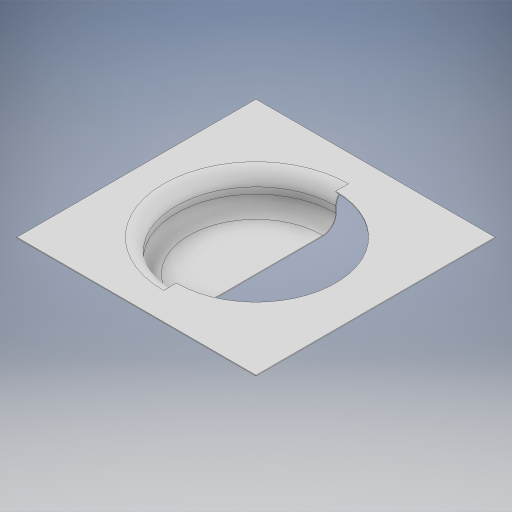
# Autodesk Inventor part: A3.2
Saved by Autodesk Inventor 2024 (Build 280153000, 153)
## iProperties
Created: 2024-03-14
Part Number: A3.2
Material: Generic
Document SubType Name: Sheet Metal
Designer: Alex
Density: 1 g/cm^3
Sheet Metal Rule: Default_mm
Appearance: Default
Author: Alex
Autodesk Inventor part; units mm, degrees
ref_plane "YZ Plane" through (0, 0, 0) normal (1, 0, 0) x (0, 1, 0)
ref_plane "XZ Plane" through (0, 0, 0) normal (0, 1, 0) x (-1, 0, 0)
sketch "Sketch1" plane through (0, 0, 0) normal (0, 1, 0) x (-1, 0, 0)
  line L0 (0, 0) -> (-150, 0)
  line L1 (-150, 0) -> (-150, -150)
  line L2 (-150, -150) -> (0, -150)
  line L3 (0, -150) -> (0, 0)
  dimension "d0" = 150
  dimension "d1" = 150
  measures "d0" distance of L2.end L1.end
  measures "d1" distance of L1.end L0.end
extrude "Plate1" add sketch "Sketch1" along normal blind 0.5
sketch "Sketch2" plane through (0, 0.5, 0) normal (0, 1, 0) x (1, 0, 0)
  arc A0 (75, 133) -> (75, 17) centre (75, 75) ccw
  line L0 (0, 0) -> (0, 150) projected
  line L1 (0, 150) -> (150, 150) projected
  line L2 (75, 17) -> (75, 133) construction
  arc A1 (75, 25) -> (75, 125) centre (75, 75) ccw
  line L3 (75, 125) -> (75, 133)
  line L4 (75, 25) -> (75, 17)
  arc A2 (75, 17) -> (75, 133) centre (75, 75) ccw construction
  dimension "d3" = 75
  dimension "d4" = 75
  dimension "d5" = 116
  dimension "d7" = 50
  constraints: 6 end point, 6 point on circle, 3 centre point, 2 coincident, 2 collinear, 2 point on line, 1 midpoint, 1 vertical
  measures "d3" distance from line of L0 A0.centre
  measures "d4" distance from line of L1 A0.centre
  measures "d5" diameter of A0
  measures "d7" radius of A1
extrude "Extrusion1" cut sketch "Sketch2" against normal blind 0.5
ref_plane "Work Plane1" through (75, 0.5, -75) normal (0, 0, -1) x (-1, 0, 0)
sketch "Sketch3" plane through (75, 0.5, -75) normal (0, 0, -1) x (-1, 0, 0)
  line L0 (58, 0) -> (0, 0) construction
  line L1 (0, 0) -> (0, -0.5) projected
  line L2 (0, 0) -> (0, -20)
  line L3 (0, -20) -> (42, -20)
  arc A0 (42, -20) -> (50, -12) centre (42, -12) ccw
  line L4 (50, -12) -> (50, -8)
  arc A1 (58, 0) -> (50, -8) centre (58, -8) ccw
  line L5 (58, 0) -> (58, -0.5)
  arc A2 (58, -0.5) -> (50.5, -8) centre (58, -8) ccw
  line L6 (50.5, -8) -> (50.5, -12)
  arc A3 (42, -20.5) -> (50.5, -12) centre (42, -12) ccw
  line L7 (42, -20.5) -> (0, -20.5)
  line L8 (0, -20.5) -> (0, -20)
  line L9 (42, -20) -> (42, -20.5) construction
  line L10 (50.5, -8) -> (50, -8) construction
  point P0 (75, -0.5)
  dimension "d10" = 20
  dimension "d12" = 8
  dimension "d13" = 8
  dimension "d14" = 0.5
  dimension "d15" = 0.5
  dimension "d16" = 0.5
  constraints: 18 end point, 8 point on circle, 7 tangent, 4 centre point, 4 perpendicular, 3 vertical, 2 horizontal
  measures "d10" distance of L1.start L2.end
  measures "d12" radius of A1
  measures "d13" radius of A0
  measures "d14" distance of L0.start L5.end
  measures "d15" distance of L7.end L2.end
  measures "d16" distance of L6.start L4.end
revolve "Revolution1" add sketch "Sketch3" angle 180 mid plane about axis through (75, 0.5, -75) along (0, -1, 0)
equation "\"d8\" = Thickness"
equation "\"d14\" = Thickness"
equation "\"d15\" = Thickness"
equation "\"d16\" = Thickness"
equation "\"d2\" = Thickness"
equation "\"BendRadius\" = Thickness"
equation "\"BendReliefWidth\" = Thickness"
equation "\"BendReliefDepth\" = 0.5 * Thickness"
equation "\"CornerReliefSize\" = 4 * Thickness"
equation "\"MinimumRemnant\" = 2 * Thickness"
equation "\"TransitionRadius\" = BendRadius"
equation "\"JacobiRadiusSize\" = BendRadius"
equation "\"GapSize\" = Thickness"
equation "\"Thickness\" = 0.5"
body "Solid1"
